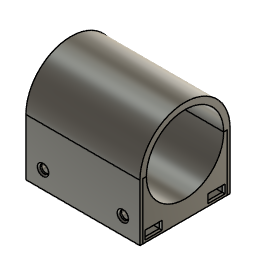
05 Powerbank v7 (Autodesk Fusion 360 design; units mm, degrees)
Autodesk Fusion 360 part; units mm, degrees
sketch "Sketch1" plane through (0, 0, 0) normal (0, 0, 1) x (1, 0, 0)
  circle A0 centre (-16, 23) radius 13.56
  line L0 (40, 14) -> (80, 14)
  line L1 (80, -15.62) -> (40, -15.62)
  line L2 (40, -15.62) -> (40, -9.34)
  line L3 (40, -15.62) -> (40, -14.34)
  line L4 (40, -14.34) -> (51, -14.34)
  line L5 (51, -14.34) -> (51, -9.34)
  line L6 (51, -9.34) -> (40, -9.34)
  line L7 (80, -15.62) -> (80, -14.34)
  line L8 (80, -14.34) -> (69, -14.34)
  line L9 (69, -14.34) -> (69, -9.34)
  line L10 (69, -9.34) -> (80, -9.34)
  line L11 (80, 14) -> (80, 12.72)
  line L12 (80, 12.72) -> (69, 12.72)
  line L13 (69, 12.72) -> (69, 7.72)
  line L14 (69, 7.72) -> (80, 7.72)
  line L15 (80, 14) -> (80, 7.72)
  line L16 (80, -9.34) -> (80, -15.62)
  line L17 (40, 14) -> (40, -9.34)
  line L18 (80, 7.72) -> (80, -9.34)
  line L19 (40, 14) -> (40, 12.72)
  line L20 (40, 12.72) -> (51, 12.72)
  line L21 (51, 12.72) -> (51, 7.72)
  line L22 (51, 7.72) -> (40, 7.72)
  line L23 (-16.5167, -20.4704) -> (-1.7067, -20.4704)
  line L24 (-16.5167, -20.4704) -> (-31.3267, -20.4704)
  arc A1 (-30.0767, -20.4704) -> (-2.9567, -20.4704) centre (-16.5167, -20.4704) ccw
  arc A2 (-32.3267, -20.4704) -> (-0.7067, -20.4704) centre (-16.5167, -20.4704) ccw
  line L25 (-32.3267, -20.4704) -> (-32.3267, -5.6304)
  line L26 (-32.3267, -5.6304) -> (-31.3267, -5.6304)
  line L27 (-31.3267, -5.6304) -> (-31.3267, -20.4704)
  line L28 (-0.7067, -20.4704) -> (-0.7067, -5.6304)
  line L29 (-0.7067, -5.6304) -> (-1.7067, -5.6304)
  line L30 (-1.7067, -5.6304) -> (-1.7067, -20.4704)
  point P0 (-16, 23)
  dimension "d1" = 27.12
  dimension "d3" = 40
  dimension "d4" = 29.62
  dimension "d5" = 1.28
  dimension "d6" = 11
  dimension "d7" = 5
  dimension "d8" = 1.28
  dimension "d9" = 11
  dimension "d10" = 5
  dimension "d23" = 1.28
  dimension "d24" = 11
  dimension "d25" = 5
  dimension "d26" = 1.28
  dimension "d27" = 11
  dimension "d28" = 5
  dimension "d49" = 14.84
  dimension "d51" = 14.84
  constraint horizontal L0
  constraint vertical L15
  constraint horizontal L1
  constraint vertical L2
  constraint perpendicular L1 L3
  constraint perpendicular L2 L4
  constraint perpendicular L4 L5
  constraint perpendicular L2 L6
  constraint perpendicular L1 L7
  constraint perpendicular L7 L8
  constraint perpendicular L8 L9
  constraint coincident L10.end L15
  constraint perpendicular L10 L15
  constraint perpendicular L0 L11
  constraint perpendicular L11 L12
  constraint perpendicular L12 L13
  constraint perpendicular L14 L15
  constraint collinear L15 L16
  constraint perpendicular L0 L17
  constraint perpendicular L0 L19
  constraint perpendicular L17 L20
  constraint perpendicular L20 L21
  constraint coincident L17 L22.end
  constraint perpendicular L17 L22
  constraint concentric A1 A2
  constraint coincident L23.start L24.start
  constraint horizontal L23
  constraint horizontal L24
  constraint coincident L23 A1.end
  constraint coincident L24 A1.start
  constraint vertical L25
  constraint horizontal L26
  constraint vertical L27
  constraint vertical L28
  constraint horizontal L29
  constraint vertical L30
  measures "d3" distance of L0.start L0.end
  measures "d4" distance of L0.start L1.end
  measures "d5" distance of L1.end L3.end
  measures "d6" distance of L3.end L4.end
  measures "d7" distance of L4.end L5.end
  measures "d8" distance of L1.start L7.end
  measures "d9" distance of L7.end L8.end
  measures "d10" distance of L8.end L9.end
  measures "d23" distance of L0.end L11.end
  measures "d24" distance of L11.end L12.end
  measures "d25" distance of L12.end L13.end
  measures "d26" distance of L0.start L19.end
  measures "d27" distance of L19.end L20.end
  measures "d28" distance of L20.end L21.end
  measures "d49" distance of L24.end L26.end
  measures "d51" distance of L23.end L29.end
extrude "Extrude4" add sketch "Sketch1" along normal blind 1.28 contours L0 L1 L2 L3 L4 L5 L6 L7 L8 L9 L10 L11 L12 L13 L14 L15 L16 L17 L18 L19 L20 L21 L22 | L17 L20 L21 L22 | L12 L13 L14 L15 | L2 L4 L5 L6 | L8 L9 L10 L16 makes body 1
extrude "Extrude5" add sketch "Sketch1" along normal blind 13.56 separate body contours L0 L1 L2 L3 L4 L5 L6 L7 L8 L9 L10 L11 L12 L13 L14 L15 L16 L17 L18 L19 L20 L21 L22 | L17 L20 L21 L22 | L12 L13 L14 L15 | L2 L4 L5 L6 | L8 L9 L10 L16 makes body 2
move_body "Move3" bodies 2 to x (1, 0, 0) y (0, 1, 0) z (0, 0, 1) at (0, 0, 1.28)
extrude "Extrude6" add sketch "Sketch1" along normal blind 40 separate body contours A0 makes body 3
move_body "Align1" bodies 3 to x (0, 1, 0) y (0, 0, 1) z (1, 0, 0) at (40, 15.19, -8.16)
combine "Combine1" operation add target body 1 tool bodies 2
combine "Combine2" operation cut target body 1 tool bodies 3
extrude "Extrude7" add sketch "Sketch1" along normal blind 2 separate body contours L17 L20 L21 L22 | L12 L13 L14 L15 | L2 L4 L5 L6 | L8 L9 L10 L16 makes body 4 at (72.6667, -11.0067, 0) makes body 5 at (72.6667, 11.0533, 0) makes body 6 at (43.6667, -11.0067, 0) makes body 7 at (43.6667, 11.0533, 0)
move_body "Move4" bodies 4 7 5 6 to x (1, 0, 0) y (0, 1, 0) z (0, 0, 1) at (0, 0, 1)
combine "Combine3" operation cut target body 1 tool bodies 4 7 5 6
extrude "Extrude10" add sketch "Sketch1" along normal blind 40 separate body contours L23 L24 A1 A2 L25 L26 L27 L28 L29 L30 makes body 8
move_body "Align4" bodies 8 to x (0, -1, 0) y (0, 0, -1) z (1, 0, 0) at (40, -17.3267, -5.6304)
chamfer "Chamfer1" distance 0.5 angle 45 8 edges at (80, -9.34, 2) (80, -11.84, 3) (80, -14.34, 2) (80, -11.84, 1) (80, 7.72, 2) (80, 10.22, 3) (80, 12.72, 2) (80, 10.22, 1) on bodies 1
chamfer "Chamfer2" distance 0.5 angle 45 8 edges at (40, 10.22, 3) (40, 12.72, 2) (40, 10.22, 1) (40, 7.72, 2) (40, -9.34, 2) (40, -11.84, 3) (40, -14.34, 2) (40, -11.84, 1) on bodies 1
move_face "MoveFace2" by (0, 0, -5) 3 faces at (53.3333, -5.7467, 0) (66.6667, -16.2867, 0) (66.6667, 14.6667, 0) on bodies 1 8
move_face "MoveFace3" by (0, 0, -4.7) 9 faces at (69, -12.6733, 1.6667) (72.5, -14.34, 2.3333) (72.5, -12.6733, 1) (72.5, -9.34, 1.6667) (72.5, -12.6733, 3) (79.8333, -12.6733, 3.3333) (79.8333, -14.6733, 2.3333) (79.8333, -12.6733, 0.6667) (79.8333, -9.0067, 1.6667) on bodies 1
move_face "MoveFace4" by (0, 0, -4.7) 9 faces at (72.5, 11.0533, 1) (69, 11.0533, 1.6667) (72.5, 7.72, 1.6667) (72.5, 11.0533, 3) (72.5, 12.72, 2.3333) (79.8333, 13.0533, 2.3333) (79.8333, 9.3867, 3.3333) (79.8333, 7.3867, 2.3333) (79.8333, 11.0533, 0.6667) on bodies 1
move_face "MoveFace5" by (0, 0, -4.7) 9 faces at (51, -12.6733, 1.6667) (44, -11.0067, 3) (44, -9.34, 2.3333) (44, -14.34, 2.3333) (44, -11.0067, 1) (40.1667, -11.0067, 3.3333) (40.1667, -14.6733, 2.3333) (40.1667, -11.0067, 0.6667) (40.1667, -9.0067, 1.6667) on bodies 1
move_face "MoveFace6" by (0, 0, -4.7) 9 faces at (51, 9.3867, 2.3333) (44, 11.0533, 3) (44, 11.0533, 1) (44, 7.72, 2.3333) (44, 12.72, 2.3333) (40.1667, 13.0533, 2.3333) (40.1667, 11.0533, 3.3333) (40.1667, 7.3867, 2.3333) (40.1667, 9.3867, 0.6667) on bodies 1
sketch "Sketch3" plane through (0, -16.62, 0) normal (0, -1, 0) x (1, 0, 0)
  line L0 (40, 14.84) -> (40, -5)
  line L1 (40, -5) -> (80, -5)
  line L2 (80, -5) -> (80, 14.84)
  line L3 (80, 14.84) -> (40, 14.84)
  line L4 (40, -5) -> (46, -5)
  line L5 (46, -5) -> (46, 1)
  circle A0 centre (46, 1) radius 1.5
  line L6 (80, -5) -> (74, -5)
  line L7 (74, -5) -> (74, 1)
  circle A1 centre (74, 1) radius 1.5
  dimension "d56" = 6
  dimension "d57" = 3
  dimension "d58" = 6
  dimension "d59" = 6
  dimension "d60" = 3
  constraint coincident L0.end L1.start
  constraint perpendicular L0 L4
  constraint perpendicular L1 L5
  constraint coincident L5.end A0.centre
  constraint coincident L1.end L2.start
  constraint perpendicular L2 L6
  constraint perpendicular L6 L7
  constraint coincident L7.end A1.centre
  measures "d56" distance of L0.end L4.end
  measures "d57" diameter of A0
  measures "d58" distance of L1.end L6.end
  measures "d59" distance of L6.end L7.end
  measures "d60" diameter of A1
extrude "Extrude11" cut sketch "Sketch3" against normal blind 7 contours A0 | A1 bodies 1 8
sketch "Sketch4" plane through (0, 15, 0) normal (0, 1, 0) x (-1, 0, 0)
  line L0 (-40, -5) -> (-40, 14.84)
  line L1 (-40, 14.84) -> (-80, 14.84)
  line L2 (-80, 14.84) -> (-80, -5)
  line L3 (-80, -5) -> (-40, -5)
  circle A0 centre (-74, 1) radius 1.5
  circle A1 centre (-46, 1) radius 1.5
  dimension "d67" = 3
  dimension "d68" = 3
  measures "d67" diameter of A0
  measures "d68" diameter of A1
extrude "Extrude12" cut sketch "Sketch4" against normal blind 7 contours A0 | A1 bodies 1 8
chamfer "Chamfer3" distance 0.5 angle 45 4 edges at (47.3985, 15, 1.5424) (75.3985, 15, 1.5424) (44.6015, -16.62, 1.5424) (72.6015, -16.62, 1.5424) on bodies 8
equation "d1 = 26.92 mm + 0.2 mm"
named bodies: "powerbank_case_bottom", "powerbank_case_top"
